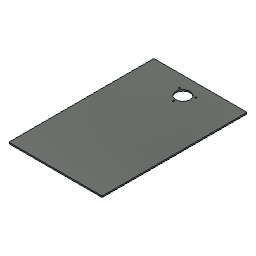
Rear Panel (x1) v3 (Autodesk Fusion 360 design; units mm, degrees)
Autodesk Fusion 360 part; units mm, degrees
sketch "Sketch1" plane through (0, 0, 0) normal (0, 0, 1) x (1, 0, 0)
  line L0 (2, 0) -> (210, 0)
  line L1 (212, 2) -> (212, 327)
  line L2 (210, 329) -> (2, 329)
  line L3 (0, 327) -> (0, 2)
  arc A0 (2, 329) -> (0, 327) centre (2, 327) ccw
  arc A1 (212, 327) -> (210, 329) centre (210, 327) ccw
  arc A2 (210, 0) -> (212, 2) centre (210, 2) ccw
  arc A3 (0, 2) -> (2, 0) centre (2, 2) ccw
  point P0 (212, 0)
  point P1 (0, 329)
  dimension "d1" = 212
  dimension "d2" = 329
  dimension "d3" = 2
  constraint horizontal L0
  constraint vertical L1
  constraint horizontal L2
  constraint vertical L3
  constraint coincident P1 L2
  constraint coincident P1 L3
  constraint tangent L2 A0
  constraint tangent L3 A0
  constraint tangent L1 A1
  constraint tangent L2 A1
  constraint equal A0 A1
  constraint coincident P0 L0
  constraint coincident P0 L1
  constraint tangent L0 A2
  constraint tangent L1 A2
  constraint equal A0 A2
  constraint coincident origin L0
  constraint coincident origin L3
  constraint tangent L0 A3
  constraint tangent L3 A3
  constraint equal A0 A3
  measures "d1" distance of origin P0
  measures "d2" distance of origin P1
  measures "d3" radius of A0
sketch "Sketch2" plane through (0, 0, 0) normal (0, 0, 1) x (1, 0, 0)
  circle A0 centre (106, 289) radius 16
  line L0 (210, 329) -> (2, 329)
  line L1 (106, 329) -> (106, 0) construction
  circle A1 centre (106, 267.5) radius 1.65
  circle A2 centre (124.6195, 299.75) radius 1.65
  circle A3 centre (87.3805, 299.75) radius 1.65
  dimension "d4" = 32
  dimension "d5" = 40
  dimension "d6" = 3.3
  dimension "d7" = 21.5
  dimension "d9" = 360
  constraint midpoint L0 L1.start
  constraint perpendicular L0 L1
  constraint coincident A0.centre L1
  constraint coincident L1 A1.centre
  measures "d4" diameter of A0
  measures "d5" distance of A0.centre L0
  measures "d6" diameter of A1
  measures "d7" distance of A0.centre A1.centre
extrude "Extrude1" add sketch "Sketch1" along normal blind 3
extrude "Extrude2" cut sketch "Sketch2" along normal blind 3
sketch "Sketch3" plane through (0, 0, 3) normal (0, 0, 1) x (-1, 0, 0)
  circle A0 centre (-87.3805, -299.75) radius 1.65
  circle A1 centre (-106, -267.5) radius 1.65
  circle A2 centre (-106, -289) radius 16
  circle A3 centre (-124.6195, -299.75) radius 1.65
  arc A4 (0, -2) -> (-2, 0) centre (-2, -2) ccw
  line L0 (-2, 0) -> (-210, 0)
  arc A5 (-210, 0) -> (-212, -2) centre (-210, -2) ccw
  line L1 (-212, -2) -> (-212, -327)
  arc A6 (-212, -327) -> (-210, -329) centre (-210, -327) ccw
  line L2 (-210, -329) -> (-2, -329)
  arc A7 (-2, -329) -> (0, -327) centre (-2, -327) ccw
  line L3 (0, -327) -> (0, -2)
equation "d7 = 3.85 mm + ( 3.3 / 2 ) * 1 mm + ( 32 / 2 ) * 1 mm"
